Autodesk Fusion 360 part; units mm, degrees
(part 2 of 2)
sketch "Sketch11" plane through (0, 6.5, 0) normal (0, 1, 0) x (-1, 0, 0)
  line L0 (-40.9, 0) -> (-40.9, -16)
  line L1 (-40.9, -16) -> (-23.901, -16)
  line L2 (-23.901, -16) -> (-16.75, -17.1541)
  line L3 (-16.75, -17.1541) -> (-16.75, -8)
  line L4 (-16.75, -8) -> (-16.75, 1.1541)
  line L5 (-16.75, 1.1541) -> (-23.901, 0)
  line L6 (-23.901, 0) -> (-40.9, 0)
  arc A0 (2.6304, -1.5907) -> (-7.7128, 2.6127) centre (-6, -8) ccw
  arc A1 (-7.7128, 2.6127) -> (-11.9178, 0.9745) centre (-6, -8) ccw
  arc A2 (-16.75, -8) -> (-7.7128, -18.6127) centre (-6, -8) ccw
  line L7 (-16.75, -8) -> (-16.75, -17.1541)
  line L8 (-16.75, -17.1541) -> (-7.7128, -18.6127)
  arc A3 (-7.7128, 2.6127) -> (-16.75, -8) centre (-6, -8) ccw
  line L9 (-7.7128, 2.6127) -> (-16.75, 1.1541)
  line L10 (-16.75, 1.1541) -> (-16.75, -8)
  line L11 (-63.1, -16) -> (-63.1, 0)
  line L12 (-63.1, 0) -> (-68.099, 0)
  line L13 (-68.099, 0) -> (-75.25, 1.1541)
  line L14 (-75.25, 1.1541) -> (-75.25, -8)
  line L15 (-75.25, -8) -> (-75.25, -17.1541)
  line L16 (-75.25, -17.1541) -> (-68.099, -16)
  line L17 (-68.099, -16) -> (-63.1, -16)
  arc A4 (-84.2872, -18.6127) -> (-75.25, -8) centre (-86, -8) ccw
  arc A5 (-84.2872, -18.6127) -> (-75.25, -8) centre (-86, -8) ccw
  line L18 (-84.2872, -18.6127) -> (-75.25, -17.1541)
  line L19 (-75.25, -17.1541) -> (-75.25, -8)
  arc A6 (-84.2872, -18.6127) -> (-84.2872, 2.6127) centre (-86, -8) ccw
  arc A7 (-84.2872, 2.6127) -> (-84.2872, -18.6127) centre (-86, -8) ccw
  circle A8 centre (-86, -8) radius 3
  arc A9 (-75.25, -8) -> (-84.2872, 2.6127) centre (-86, -8) ccw
  line L20 (-75.25, -8) -> (-75.25, 1.1541)
  line L21 (-75.25, 1.1541) -> (-84.2872, 2.6127)
  circle A10 centre (-52, -12) radius 1.75
  circle A11 centre (-52, -4) radius 1.75
  line L22 (-47.9, -16) -> (-47.9, 0)
  line L23 (-47.9, 0) -> (-56.1, 0)
  line L24 (-56.1, 0) -> (-56.1, -16)
  line L25 (-56.1, -16) -> (-47.9, -16)
  line L26 (-60.1, -16) -> (-56.1, -16)
  line L27 (-56.1, -16) -> (-56.1, 0)
  line L28 (-56.1, 0) -> (-60.1, 0)
  line L29 (-60.1, 0) -> (-60.1, -16)
  line L30 (-63.1, -16) -> (-60.1, -16)
  line L31 (-60.1, -16) -> (-60.1, 0)
  line L32 (-60.1, 0) -> (-63.1, 0)
  line L33 (-63.1, 0) -> (-63.1, -16)
  line L34 (-47.9, -16) -> (-43.9, -16)
  line L35 (-43.9, -16) -> (-43.9, 0)
  line L36 (-43.9, 0) -> (-47.9, 0)
  line L37 (-47.9, 0) -> (-47.9, -16)
  line L38 (-40.9, 0) -> (-43.9, 0)
  line L39 (-43.9, 0) -> (-43.9, -16)
  line L40 (-43.9, -16) -> (-40.9, -16)
  line L41 (-40.9, -16) -> (-40.9, 0)
  line L42 (-6, -8) -> (-86, -8) construction
  line L43 (-22.325, -4.5) -> (-35.325, -4.5)
  arc A12 (-35.325, -4.5) -> (-35.325, -11.5) centre (-35.325, -8) ccw
  line L44 (-35.325, -11.5) -> (-22.325, -11.5)
  arc A13 (-22.325, -11.5) -> (-22.325, -4.5) centre (-22.325, -8) ccw
  line L45 (-22.325, -8) -> (-35.325, -8) construction
  line L46 (-68.175, -4.5) -> (-70.175, -4.5)
  arc A14 (-70.175, -4.5) -> (-70.175, -11.5) centre (-70.175, -8) ccw
  line L47 (-70.175, -11.5) -> (-68.175, -11.5)
  arc A15 (-68.175, -11.5) -> (-68.175, -4.5) centre (-68.175, -8) ccw
  line L48 (-68.175, -8) -> (-70.175, -8) construction
  arc A16 (-3.2196, -12.4938) -> (-1.2418, -15.3184) centre (-1.985, -13.7341) ccw
  arc A17 (-3.7269, -6.0422) -> (-7.4664, -5.3828) centre (-6, -8) ccw
  arc A18 (-11.7648, -13.7648) -> (-9.9843, -11.9843) centre (-10.015, -13.7341) ccw
  arc A19 (-0.2352, -2.2352) -> (-2.0157, -4.0157) centre (-1.985, -2.2659) ccw
  arc A20 (-8.7804, -3.5062) -> (-10.7582, -0.6816) centre (-10.015, -2.2659) ccw
  circle A21 centre (-93, -8) radius 1.75
  circle A22 centre (-86, -1) radius 1.75
  circle A23 centre (-86, -15) radius 1.75
  circle A24 centre (-79, -8) radius 1.75
  line L49 (-8.7804, -3.5062) -> (-7.4664, -5.3828)
  line L50 (-3.7269, -6.0422) -> (-1.8503, -4.7281)
  arc A25 (-2.0157, -4.0157) -> (-1.8503, -4.7281) centre (-0.2659, -3.985) ccw
  arc A26 (0.9743, -2.7503) -> (-0.2352, -2.2352) centre (-0.2659, -3.985) ccw
  line L51 (0.9743, -2.7503) -> (2.6304, -1.5907)
  line L52 (-11.9178, 0.9745) -> (-10.7582, -0.6816)
  arc A27 (-7.7128, -18.6127) -> (-0.0822, -16.9745) centre (-6, -8) ccw
  line L53 (-0.0822, -16.9745) -> (-1.2418, -15.3184)
  line L54 (-3.2196, -12.4938) -> (-4.5336, -10.6172)
  arc A28 (-8.2731, -9.9578) -> (-4.5336, -10.6172) centre (-6, -8) ccw
  line L55 (-8.2731, -9.9578) -> (-10.1497, -11.2719)
  arc A29 (-9.9843, -11.9843) -> (-10.1497, -11.2719) centre (-11.7341, -12.015) ccw
  arc A30 (-12.9743, -13.2497) -> (-11.7648, -13.7648) centre (-11.7341, -12.015) ccw
  line L56 (-12.9743, -13.2497) -> (-14.6304, -14.4093)
  arc A31 (-14.6304, -14.4093) -> (-7.7128, -18.6127) centre (-6, -8) ccw
  dimension "d45" = 13
  dimension "d46" = 3.5
  dimension "d47" = 24.15
  dimension "d48" = 5.575
  dimension "d49" = 3.5
  dimension "d50" = 2
  dimension "d51" = 12.15
  dimension "d52" = 5.075
  constraint coincident A0.centre A1.centre
  constraint coincident A4.centre A5.centre
  constraint tangent L43 A12
  constraint tangent A12 L44
  constraint parallel L43 L44
  constraint tangent L44 A13
  constraint tangent L43 A13
  constraint coincident L42 A12.centre
  constraint parallel L42 L45
  constraint tangent L46 A14
  constraint tangent A14 L47
  constraint parallel L46 L47
  constraint tangent L47 A15
  constraint tangent L46 A15
  constraint coincident L42 A14.centre
  constraint perpendicular L22 L48
  measures "d45" distance of A13.centre A12.centre
  measures "d46" distance of A13.centre L44
  measures "d47" distance of L10 L41
  measures "d48" distance of L4 A13.centre
  measures "d49" distance of A15.centre L46
  measures "d50" distance of A15.centre A14.centre
  measures "d51" distance of L11 L20
  measures "d52" distance of L14.end A14.centre
extrude "Extrude11" cut sketch "Sketch11" against normal up to surface (6.5 mm away) contours L43 A12 L44 A13 | L46 A14 L47 A15
fillet "Fillet1" radius 0.5 8 edges at (28.825, 6.5, -4.5) (18.825, 6.5, -8) (28.825, 6.5, -11.5) (38.825, 6.5, -8) (69.175, 6.5, -4.5) (64.675, 6.5, -8) (69.175, 6.5, -11.5) (73.675, 6.5, -8)
chamfer "Chamfer2" distance 0.5 angle 45 18 edges at (20.3255, 6.5, 0.5771) (32.4005, 6.5, 0) (42.4, 8, 0) (45.9, 9.5, 0) (47.9, 9.5, -8) (45.9, 9.5, -16) (42.4, 8, -16) (32.4005, 6.5, -16) (20.3255, 6.5, -16.5771) (56.1, 9.5, -8) (58.1, 9.5, 0) (61.6, 8, 0) (65.5995, 6.5, 0) (71.6745, 6.5, 0.5771) (71.6745, 6.5, -16.5771) (65.5995, 6.5, -16) (61.6, 8, -16) (58.1, 9.5, -16)
chamfer "Chamfer3" distance 0.5 angle 45 6 edges at (47.9, 7.5, 0) (52, 6, 0) (56.1, 7.5, 0) (47.9, 7.5, -16) (52, 6, -16) (56.1, 7.5, -16)
chamfer "Chamfer4" distance 0.5 angle 45 8 edges at (46, 0, 0) (15.8069, 0, 1.3063) (15.8069, 0, -17.3063) (-4.75, 0, -8) (46, 0, -16) (76.1931, 0, 1.3063) (76.1931, 0, -17.3063) (96.75, 0, -8)
equation "d30 = d29 / 2"
equation "d39 = d38"
equation "d41 = d42 / 4"
equation "d48 = ( d47 - d45 ) / 2"
equation "d49 = d46"
equation "d52 = ( d51 - d50 ) / 2"
equation "d65 = d60"
equation "d66 = d61"

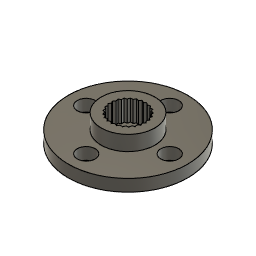
design "25TServoHorn"
Autodesk Fusion 360 part; units mm, degrees
sketch "Sketch1" plane through (0, 0, 0) normal (0, 1, 0) x (1, 0, 0)
  circle A0 centre (0, 0) radius 10
  circle A1 centre (0, 0) radius 4.5
  circle A2 centre (0, 0) radius 2.75
  circle A3 centre (0, 0) radius 1.5
  dimension "d1" = 20
  dimension "d2" = 9
  dimension "d3" = 5.5
  dimension "d4" = 3
  constraint coincident A0.centre A1.centre
  constraint concentric A1 A2
  measures "d1" diameter of A0
  measures "d2" diameter of A1
  measures "d3" diameter of A2
  measures "d4" diameter of A3
extrude "Extrude1" add sketch "Sketch1" along normal blind 2 contours A0
extrude "Extrude2" add sketch "Sketch1" along normal blind 4.5 contours A1
extrude "Extrude3" add sketch "Sketch1" along normal blind 1 contours A2
sketch "Sketch2" plane through (0, 2, 0) normal (0, 1, 0) x (-1, 0, 0)
  circle A0 centre (0, 0) radius 4.5
  circle A1 centre (0, 0) radius 10
  circle A2 centre (0, 0) radius 7
  circle A3 centre (7, 0) radius 1.5
  line L0 (0, 0) -> (10, 0) construction
  dimension "d11" = 14
  dimension "d12" = 3
  constraint concentric A0 A2
  constraint coincident A2 A3.centre
  constraint coincident A0.centre A1.centre
  constraint coincident A1 L0.end
  constraint horizontal L0
  constraint coincident A3.centre L0
  measures "d11" diameter of A2
  measures "d12" diameter of A3
extrude "Extrude4" cut sketch "Sketch2" against normal up to surface (2 mm away) contours A2 A3 | A2 A3 picked at (6.5153, -0.3111) picked at (7.4507, -0.3705)
pattern_circular "C-Pattern1" count 4 over 360 about axis through (0, 1.75, 0) along (0, 1, 0) of "Extrude4"
sketch "Sketch3" plane through (0, 4.5, 0) normal (0, 1, 0) x (-1, 0, 0)
  circle A0 centre (0, 0) radius 2.75
  circle A1 centre (0, 0) radius 4.5
  circle A2 centre (0, 0) radius 3
  line L0 (0, 0) -> (3, 0)
  line L1 (0, 0) -> (2.9763, -0.376)
  line L2 (0, 0) -> (2.9057, -0.7461)
  line L3 (2.6636, -0.6839) -> (2.9763, -0.376)
  line L4 (2.75, 0) -> (2.9763, -0.376)
  dimension "d17" = 6
  dimension "d18" = 7.2
  dimension "d19" = 14.4
  constraint concentric A0 A2
  constraint coincident A0.centre A1.centre
  constraint coincident A2 L0.end
  constraint horizontal L0
  constraint coincident A2 L1.end
  constraint coincident A2 L2.end
  constraint coincident L2 L3.start
  constraint coincident A0 L3.start
  constraint coincident L0 L4.start
  constraint coincident A0 L4.start
  measures "d17" diameter of A2
  measures "d18" angle of L0 L1
  measures "d19" angle of L0 L2
extrude "Extrude5" cut sketch "Sketch3" against normal up to surface (3.5 mm away) contours A0 L1 L4 | A0 L1 L3
pattern_circular "C-Pattern2" count 25 over 360 about axis through (0, 1.75, 0) along (0, 1, 0) of "Extrude5"

design "FrameSideServoHolder"
Autodesk Fusion 360 part; units mm, degrees
sketch "Sketch1" plane through (0, 0, 0) normal (0, 1, 0) x (1, 0, 0)
  line L0 (0, 0) -> (0, 7)
  line L1 (0, 7) -> (19, 7)
  line L2 (19, 7) -> (19, 48)
  line L3 (19, 48) -> (0, 48)
  line L4 (0, 48) -> (0, 55)
  line L5 (0, 55) -> (25, 55)
  line L6 (25, 55) -> (25, 34.5)
  line L7 (25, 34.5) -> (34.8, 24.7)
  line L8 (34.8, 24.7) -> (34.8, -3.9005)
  line L9 (34.8, -3.9005) -> (29.8503, -8.8503)
  line L10 (0, 0) -> (21, 0)
  line L11 (21, 0) -> (29.8503, -8.8503)
  line L12 (0, 7) -> (23.8995, 7) construction
  line L13 (23.8995, 7) -> (34.8, -3.9005) construction
  dimension "d1" = 7
  dimension "d2" = 7
  dimension "d3" = 19
  dimension "d4" = 41
  dimension "d5" = 135
  dimension "d6" = 6
  dimension "d7" = 20.5
  dimension "d8" = 15.8
  dimension "d9" = 135
  dimension "d10" = 7
  dimension "d11" = 2
  dimension "d12" = 7
  constraint coincident L0.start L10.start
  constraint vertical L0
  constraint perpendicular L0 L1
  constraint perpendicular L1 L2
  constraint perpendicular L0 L3
  constraint perpendicular L3 L4
  constraint perpendicular L4 L5
  constraint perpendicular L5 L6
  constraint vertical L8
  constraint perpendicular L0 L10
  constraint collinear L0 L4
  constraint perpendicular L9 L11
  constraint coincident L0 L1.start
  constraint perpendicular L0 L12
  constraint parallel L11 L13
  measures "d1" distance of L0.start L0.end
  measures "d2" distance of L3.end L4.end
  measures "d3" distance of L2 L4
  measures "d4" distance of L1.end L2.end
  measures "d5" angle of L6 L7
  measures "d6" distance of L2 L6
  measures "d7" distance of L5.end L6.end
  measures "d8" distance of L2 L8
  measures "d9" angle of L10 L11
  measures "d10" distance of L8.end L9.end
  measures "d11" distance of L2 L10.end
  measures "d12" distance of L10 L12
extrude "Extrude1" add sketch "Sketch1" along normal blind 16
sketch "Sketch2" plane through (0, 16, 0) normal (0, 1, 0) x (-1, 0, 0)
  line L0 (0, 0) -> (-21, 0)
  line L1 (-21, 0) -> (-29.8503, 8.8503)
  line L2 (-29.8503, 8.8503) -> (-34.8, 3.9005)
  line L3 (-34.8, 3.9005) -> (-34.8, -24.7)
  line L4 (-34.8, -24.7) -> (-25, -34.5)
  line L5 (-25, -34.5) -> (-25, -55)
  line L6 (-25, -55) -> (0, -55)
  line L7 (0, -55) -> (0, -48)
  line L8 (0, -48) -> (-19, -48)
  line L9 (-19, -48) -> (-19, -7)
  line L10 (-19, -7) -> (0, -7)
  line L11 (0, -7) -> (0, 0)
  line L12 (-4.5, -51.5) -> (-14.5, -51.5) construction
  line L13 (-14.5, -51.5) -> (-14.5, -3.5) construction
  line L14 (-14.5, -3.5) -> (-4.5, -3.5) construction
  line L15 (-4.5, -3.5) -> (-4.5, -51.5) construction
  circle A0 centre (-4.5, -51.5) radius 1.75
  circle A1 centre (-14.5, -51.5) radius 1.75
  circle A2 centre (-14.5, -3.5) radius 1.75
  circle A3 centre (-4.5, -3.5) radius 1.75
  dimension "d15" = 10
  dimension "d16" = 48
  dimension "d17" = 19
  dimension "d18" = 55
  dimension "d19" = 3.5
  dimension "d20" = 4.5
  dimension "d21" = 3.5
  dimension "d22" = 3.5
  dimension "d23" = 3.5
  dimension "d24" = 3.5
  constraint horizontal L12
  constraint vertical L13
  constraint horizontal L14
  constraint vertical L15
  constraint coincident L12.start L15.end
  constraint coincident L12.end L13.start
  constraint coincident L13.end L14.start
  constraint coincident L14.end L15.start
  measures "d15" distance of L12.start L12.end
  measures "d16" distance of L12.start L14.end
  measures "d17" distance of L7 L9
  measures "d18" distance of L0 L6
  measures "d19" distance of L6 L12
  measures "d20" distance of L7 L15
  measures "d21" diameter of A0
  measures "d22" diameter of A1
  measures "d23" diameter of A3
  measures "d24" diameter of A2
extrude "Extrude2" cut sketch "Sketch2" against normal up to surface (16 mm away) contours A0 | A1 | A2 | A3
sketch "Sketch3" plane through (0, 16, 0) normal (0, 1, 0) x (-1, 0, 0)
  circle A0 centre (-14.5, -51.5) radius 1.75
  circle A1 centre (-4.5, -3.5) radius 1.75
  circle A2 centre (-4.5, -51.5) radius 1.75
  circle A3 centre (-14.5, -3.5) radius 1.75
  line L0 (0, 0) -> (-21, 0)
  line L1 (-21, 0) -> (-29.8503, 8.8503)
  line L2 (-29.8503, 8.8503) -> (-34.8, 3.9005)
  line L3 (-34.8, 3.9005) -> (-34.8, -24.7)
  line L4 (-34.8, -24.7) -> (-25, -34.5)
  line L5 (-25, -34.5) -> (-25, -55)
  line L6 (-25, -55) -> (0, -55)
  line L7 (0, -55) -> (0, -48)
  line L8 (0, -48) -> (-19, -48)
  line L9 (-19, -48) -> (-19, -7)
  line L10 (-19, -7) -> (0, -7)
  line L11 (0, -7) -> (0, 0)
  line L12 (-25, -28.8431) -> (-30.8, -23.0431)
  line L13 (-25, -5.8995) -> (-25, -28.8431)
  line L14 (-30.8, -23.0431) -> (-30.8, -0.0995)
  line L15 (-30.8, -0.0995) -> (-25, -5.8995)
  dimension "d27" = 4
  dimension "d31" = 4
  dimension "d32" = 7
  constraint parallel L4 L12
  constraint parallel L9 L13
  constraint collinear L5 L13
  constraint parallel L3 L14
  constraint parallel L1 L15
  measures "d27" distance of L4 L12
  measures "d31" distance of L3 L14
  measures "d32" distance of L1 L15
extrude "Extrude3" cut sketch "Sketch3" against normal up to surface (16 mm away) contours L12 L13 L14 L15
sketch "Sketch4" plane through (0, 0, -55) normal (0, 0, -1) x (-1, 0, 0)
  line L0 (-25, 0) -> (0, 0)
  line L1 (0, 0) -> (0, 16)
  line L2 (0, 16) -> (-25, 16)
  line L3 (-25, 16) -> (-25, 0)
  line L4 (-34.8, 0) -> (-25, 0)
  line L5 (-25, 0) -> (-25, 16)
  line L6 (-25, 16) -> (-34.8, 16)
  line L7 (-34.8, 16) -> (-34.8, 0)
  line L8 (-25, 3) -> (-30, 3)
  line L9 (-30, 3) -> (-30, 13)
  line L10 (-30, 13) -> (-25, 13)
  line L11 (-25, 13) -> (-25, 3)
  dimension "d35" = 5
  dimension "d36" = 10
  dimension "d37" = 16
  dimension "d38" = 3
  constraint horizontal L8
  constraint vertical L9
  constraint horizontal L10
  constraint vertical L11
  constraint coincident L3 L8.start
  measures "d35" distance of L8.start L8.end
  measures "d36" distance of L8.end L9.end
  measures "d37" distance of L4.start L6.end
  measures "d38" distance of L4 L8
extrude "Extrude4" cut sketch "Sketch4" along normal up to surface contours L3 L5 L8 L9 L10 L11 end surface through (25, 16, -28.8431) normal (-0.707107, 0, 0.707107) offset 0
ref_plane "WorkPlane1" through (17.4, 8, -23.0749) normal (0, -1, 0) x (-1, 0, 0)
ref_plane "WorkPlane2" through (10.5, 8, -27.5) normal (0, 0, 1) x (1, 0, 0)
sketch "Sketch5" plane through (17.4, 8, -23.0749) normal (0, -1, 0) x (1, 0, 0)
  line L0 (13.4, 22.9754) -> (7.6, 17.1754)
  line L1 (7.6, 17.1754) -> (7.6, -5.7683)
  line L2 (7.6, -5.7683) -> (13.4, 0.0317)
  line L3 (13.4, 0.0317) -> (13.4, 22.9754)
  circle A0 centre (-2.9, -28.4251) radius 1.75
  circle A1 centre (-12.9, 19.5749) radius 1.75
  circle A2 centre (-12.9, -28.4251) radius 1.75
  circle A3 centre (-2.9, 19.5749) radius 1.75
  line L4 (-17.4, 23.0749) -> (3.6, 23.0749)
  line L5 (3.6, 23.0749) -> (12.4503, 31.9251)
  line L6 (12.4503, 31.9251) -> (17.4, 26.9754)
  line L7 (17.4, 26.9754) -> (17.4, -1.6251)
  line L8 (17.4, -1.6251) -> (7.6, -11.4251)
  line L9 (7.6, -11.4251) -> (7.6, -31.9251)
  line L10 (7.6, -31.9251) -> (-17.4, -31.9251)
  line L11 (-17.4, -31.9251) -> (-17.4, -24.9251)
  line L12 (-17.4, -24.9251) -> (1.6, -24.9251)
  line L13 (1.6, -24.9251) -> (1.6, 16.0749)
  line L14 (1.6, 16.0749) -> (-17.4, 16.0749)
  line L15 (-17.4, 16.0749) -> (-17.4, 23.0749)
  line L16 (7.6, 17.1754) -> (4.4518, 23.9267)
  line L17 (-0.6679, 23.0749) -> (7.6, 5.3444)
  dimension "d48" = 5
  dimension "d49" = 65
  constraint coincident L0.end L1.start
  constraint coincident L5 L16.end
  constraint coincident L4 L17.start
  constraint coincident L1 L17.end
  constraint parallel L16 L17
  measures "d48" distance of L16 L17
  measures "d49" angle of L4 L17
extrude "Extrude5" cut sketch "Sketch5" along normal mid plane 10 contours L1 L4 L5 L16 L17
sketch "Sketch6" plane through (10.5, 0, -10.5) normal (-0.707107, 0, 0.707107) x (0.707107, 0, 0.707107)
  line L0 (16.0539, 3) -> (14.8492, 3)
  line L1 (14.8492, 3) -> (14.8492, 0)
  line L2 (14.8492, 0) -> (27.3654, 0)
  line L3 (27.3654, 0) -> (27.3654, 16)
  line L4 (27.3654, 16) -> (14.8492, 16)
  line L5 (14.8492, 16) -> (14.8492, 13)
  line L6 (14.8492, 13) -> (16.0539, 13)
  line L7 (16.0539, 13) -> (16.0539, 3)
  line L8 (21.7085, 0) -> (13.5061, 0)
  line L9 (13.5061, 0) -> (13.5061, 3)
  line L10 (13.5061, 3) -> (13.5061, 13)
  line L11 (13.5061, 13) -> (13.5061, 16)
  line L12 (13.5061, 16) -> (21.7085, 16)
  line L13 (21.7085, 16) -> (21.7085, 0)
  line L14 (21.1073, 16) -> (21.1073, 0) construction
  line L15 (27.3654, 8) -> (13.5061, 8) construction
  circle A0 centre (21.1073, 8) radius 1.75
  dimension "d50" = 3.5
  constraint midpoint L4 L14.start
  constraint midpoint L2 L14.end
  constraint midpoint L3 L15.start
  constraint midpoint L10 L15.end
  constraint midpoint L14 A0.centre
  measures "d50" diameter of A0
extrude "Extrude6" cut sketch "Sketch6" against normal up to surface (7 mm away) contours L13 A0 | L13 A0
sketch "Sketch7" plane through (15.4497, 0, -15.4497) normal (0.707107, 0, -0.707107) x (-0.707107, 0, -0.707107)
  arc A0 (-21.7085, 6.3565) -> (-21.7085, 9.6435) centre (-21.1073, 8) ccw
  line L0 (-21.7085, 6.3565) -> (-21.7085, 0)
  line L1 (-21.7085, 0) -> (-13.5061, 0)
  line L2 (-13.5061, 0) -> (-13.5061, 3)
  line L3 (-13.5061, 3) -> (-13.5061, 13)
  line L4 (-13.5061, 13) -> (-13.5061, 16)
  line L5 (-13.5061, 16) -> (-21.7085, 16)
  line L6 (-21.7085, 16) -> (-21.7085, 9.6435)
  line L7 (-27.3654, 0) -> (-7.1418, 0)
  line L8 (-7.1418, 0) -> (-7.1418, 16)
  line L9 (-7.1418, 16) -> (-27.3654, 16)
  line L10 (-27.3654, 16) -> (-27.3654, 0)
  circle A1 centre (-21.1073, 8) radius 1.75
  circle A2 centre (-21.1073, 8) radius 3
  dimension "d53" = 6
  constraint concentric A0 A2
  measures "d53" diameter of A2
extrude "Extrude7" cut sketch "Sketch7" along normal up to surface contours A0 A1 | A0 L0 L6 A1 A2 | L0 L6 A1 A2 end surface through (34.8, 0, -24.7) normal (1, 0, 0) offset 0
sketch "Sketch8" plane through (17.4, 8, -23.0749) normal (0, -1, 0) x (1, 0, 0)
  line L0 (13.4, 22.9754) -> (7.6, 17.1754)
  line L1 (7.6, 17.1754) -> (7.6, -5.7683)
  line L2 (7.6, -5.7683) -> (13.4, 0.0317)
  line L3 (13.4, 0.0317) -> (13.4, 22.9754)
  circle A0 centre (-2.9, -28.4251) radius 1.75
  circle A1 centre (-12.9, 19.5749) radius 1.75
  circle A2 centre (-12.9, -28.4251) radius 1.75
  circle A3 centre (-2.9, 19.5749) radius 1.75
  line L4 (-17.4, 23.0749) -> (3.6, 23.0749)
  line L5 (3.6, 23.0749) -> (12.4503, 31.9251)
  line L6 (12.4503, 31.9251) -> (17.4, 26.9754)
  line L7 (17.4, 26.9754) -> (17.4, -1.6251)
  line L8 (17.4, -1.6251) -> (7.6, -11.4251)
  line L9 (7.6, -11.4251) -> (7.6, -31.9251)
  line L10 (7.6, -31.9251) -> (-17.4, -31.9251)
  line L11 (-17.4, -31.9251) -> (-17.4, -24.9251)
  line L12 (-17.4, -24.9251) -> (1.6, -24.9251)
  line L13 (1.6, -24.9251) -> (1.6, 16.0749)
  line L14 (1.6, 16.0749) -> (-17.4, 16.0749)
  line L15 (-17.4, 16.0749) -> (-17.4, 23.0749)
  line L16 (-10.2, 21.1337) -> (-12.9, 22.6926)
  line L17 (-12.9, 22.6926) -> (-15.6, 21.1337)
  line L18 (-15.6, 21.1337) -> (-15.6, 18.016)
  line L19 (-15.6, 18.016) -> (-12.9, 16.4572)
  line L20 (-12.9, 16.4572) -> (-10.2, 18.016)
  line L21 (-10.2, 18.016) -> (-10.2, 21.1337)
  line L22 (-0.2, 21.1337) -> (-2.9, 22.6926)
  line L23 (-2.9, 22.6926) -> (-5.6, 21.1337)
  line L24 (-5.6, 21.1337) -> (-5.6, 18.016)
  line L25 (-5.6, 18.016) -> (-2.9, 16.4572)
  line L26 (-2.9, 16.4572) -> (-0.2, 18.016)
  line L27 (-0.2, 18.016) -> (-0.2, 21.1337)
  line L28 (-15.6, 18.016) -> (-15.6, 16.0749)
  line L29 (-10.2, 18.016) -> (-10.2, 16.0749)
  line L30 (-15.6, 21.1337) -> (-15.6, 23.0749)
  line L31 (-10.2, 21.1337) -> (-10.2, 23.0749)
  line L32 (-5.6, 21.1337) -> (-5.6, 23.0749)
  line L33 (-0.2, 21.1337) -> (-0.2, 23.0749)
  line L34 (-5.6, 18.016) -> (-5.6, 16.0749)
  line L35 (-0.2, 18.016) -> (-0.2, 16.0749)
  point P0 (-12.9, 19.5749)
  point P1 (-2.9, 19.5749)
  dimension "d56" = 5.4
  dimension "d57" = 5.4
  constraint coincident P0 A1.centre
  constraint coincident P1 A3.centre
  constraint parallel L15 L18
  constraint parallel L21 L24
  constraint coincident L14 L28.end
  constraint perpendicular L14 L28
  constraint coincident L14 L29.end
  constraint perpendicular L14 L29
  constraint coincident L4 L30.end
  constraint perpendicular L4 L30
  constraint coincident L4 L31.end
  constraint perpendicular L4 L31
  constraint coincident L4 L32.end
  constraint perpendicular L4 L32
  constraint coincident L4 L33.end
  constraint perpendicular L4 L33
  constraint coincident L14 L34.end
  constraint perpendicular L14 L34
  constraint coincident L14 L35.end
  constraint perpendicular L14 L35
  measures "d56" distance of L18 L21
  measures "d57" distance of L24 L27
extrude "Extrude8" cut sketch "Sketch8" along normal mid plane 2.5 contours L4 L16 L17 L30 L31 | L16 L17 L18 L19 L20 L21 | L14 L19 L20 L28 L29 | L4 L22 L23 L32 L33 | L22 L23 L24 L25 L26 L27 | L14 L25 L26 L34 L35
mirror "Mirror1" about plane through (10.5, 8, -27.5) normal (0, 0, 1) of "Extrude8"
sketch "Sketch9" plane through (0, 0, 0) normal (0, 0, 1) x (1, 0, 0)
  line L0 (1.8, 9.25) -> (7.2, 9.25)
  line L1 (7.2, 9.25) -> (7.2, 6.75)
  line L2 (16.7321, 6.75) -> (11.8, 6.75)
  line L3 (1.8, 6.75) -> (1.8, 9.25)
  line L4 (11.8, 9.25) -> (16.7321, 9.25)
  line L5 (11.8, 6.75) -> (11.8, 9.25)
  line L6 (21, 3) -> (16.7321, 3)
  line L7 (16.7321, 9.25) -> (16.7321, 13)
  line L8 (16.7321, 13) -> (21, 13)
  line L9 (21, 13) -> (21, 16)
  line L10 (21, 16) -> (0, 16)
  line L11 (0, 16) -> (0, 0)
  line L12 (0, 0) -> (21, 0)
  line L13 (21, 0) -> (21, 3)
  line L14 (7.2, 9.25) -> (1.8, 9.25)
  line L15 (1.8, 9.25) -> (1.8, 6.75)
  line L16 (1.8, 6.75) -> (7.2, 6.75)
  line L17 (7.2, 6.75) -> (7.2, 9.25)
  line L18 (17.2, 9.25) -> (11.8, 9.25)
  line L19 (11.8, 9.25) -> (11.8, 6.75)
  line L20 (11.8, 6.75) -> (17.2, 6.75)
  line L21 (17.2, 6.75) -> (17.2, 9.25)
  line L22 (19, 0) -> (0, 0)
  line L23 (0, 0) -> (0, 16)
  line L24 (0, 16) -> (19, 16)
  line L25 (19, 16) -> (19, 0)
  line L26 (2.75, 16) -> (6.25, 16)
  line L27 (12.75, 16) -> (16.25, 16)
  line L28 (9.5, 16) -> (9.5, -0.0004) construction
  circle A0 centre (9.5, 12) radius 1.75
  circle A1 centre (9.5, 4) radius 1.75
  line L29 (16.7321, 3) -> (16.7321, 6.75)
  line L30 (7.2, 6.75) -> (1.8, 6.75)
  dimension "d60" = 19
  dimension "d61" = 9.5
  dimension "d62" = 3.5
  dimension "d63" = 3.5
  dimension "d64" = 4
  dimension "d65" = 4
  constraint vertical L28
  constraint coincident L24 L28.start
  constraint coincident L28 A0.centre
  constraint coincident L28 A1.centre
  measures "d60" distance of L11 L25
  measures "d61" distance of L23 L28
  measures "d62" diameter of A0
  measures "d63" diameter of A1
  measures "d64" distance of L24 A0.centre
  measures "d65" distance of L22 A1.centre
extrude "Extrude9" cut sketch "Sketch9" against normal up to surface (7 mm away) contours A0 | A1
sketch "Sketch10" plane through (0, 0, -7) normal (0, 0, -1) x (-1, 0, 0)
  circle A0 centre (-9.5, 12) radius 1.75
  circle A1 centre (-9.5, 4) radius 1.75
  line L0 (-7.2, 9.25) -> (-1.8, 9.25)
  line L1 (-1.8, 9.25) -> (-1.8, 6.75)
  line L2 (-1.8, 6.75) -> (-7.2, 6.75)
  line L3 (-7.2, 6.75) -> (-7.2, 9.25)
  line L4 (-17.2, 9.25) -> (-11.8, 9.25)
  line L5 (-11.8, 9.25) -> (-11.8, 6.75)
  line L6 (-11.8, 6.75) -> (-17.2, 6.75)
  line L7 (-17.2, 6.75) -> (-17.2, 9.25)
  line L8 (-19, 0) -> (0, 0)
  line L9 (0, 0) -> (0, 16)
  line L10 (0, 16) -> (-19, 16)
  line L11 (-19, 16) -> (-19, 0)
  circle A2 centre (-9.5, 12) radius 2.9
  circle A3 centre (-9.5, 4) radius 2.9
  dimension "d70" = 5.8
  dimension "d71" = 5.8
  constraint concentric A0 A2
  constraint concentric A1 A3
  measures "d70" diameter of A2
  measures "d71" diameter of A3
extrude "Extrude10" cut sketch "Sketch10" against normal blind 3 contours A2 | A3
sketch "Sketch11" plane through (0, 0, -55) normal (0, 0, -1) x (-1, 0, 0)
  line L0 (-7.2, 9.25) -> (-1.8, 9.25)
  line L1 (-1.8, 9.25) -> (-1.8, 6.75)
  line L2 (-1.8, 6.75) -> (-7.2, 6.75)
  line L3 (-7.2, 6.75) -> (-7.2, 9.25)
  line L4 (-17.2, 9.25) -> (-11.8, 9.25)
  line L5 (-11.8, 9.25) -> (-11.8, 6.75)
  line L6 (-11.8, 6.75) -> (-17.2, 6.75)
  line L7 (-17.2, 6.75) -> (-17.2, 9.25)
  line L8 (-25, 0) -> (0, 0)
  line L9 (0, 0) -> (0, 16)
  line L10 (0, 16) -> (-25, 16)
  line L11 (-25, 16) -> (-25, 0)
  circle A0 centre (-9.5, 12) radius 2.9
  circle A1 centre (-9.5, 4) radius 2.9
  line L12 (-7.2, 9.25) -> (-1.8, 9.25)
  line L13 (-1.8, 9.25) -> (-1.8, 6.75)
  line L14 (-1.8, 6.75) -> (-7.2, 6.75)
  line L15 (-7.2, 6.75) -> (-7.2, 9.25)
  line L16 (-17.2, 9.25) -> (-11.8, 9.25)
  line L17 (-11.8, 9.25) -> (-11.8, 6.75)
  line L18 (-11.8, 6.75) -> (-17.2, 6.75)
  line L19 (-17.2, 6.75) -> (-17.2, 9.25)
  line L20 (-19, 0) -> (0, 0)
  line L21 (0, 0) -> (0, 16)
  line L22 (0, 16) -> (-19, 16)
  line L23 (-19, 16) -> (-19, 0)
  circle A2 centre (-9.5, 12) radius 1.75
  circle A3 centre (-9.5, 4) radius 1.75
  circle A4 centre (-9.5, 12) radius 2.5
  circle A5 centre (-9.5, 4) radius 2.5
  dimension "d74" = 5
  dimension "d75" = 5
  constraint concentric A0 A4
  constraint concentric A3 A5
  measures "d74" diameter of A4
  measures "d75" diameter of A5
extrude "Extrude11" cut sketch "Sketch11" against normal up to surface (7 mm away) contours A2 | A3 | A4 | A5
sketch "Sketch12" plane through (0, 0, -55) normal (0, 0, -1) x (-1, 0, 0)
  circle A0 centre (-9.5, 12) radius 2.5
  circle A1 centre (-9.5, 4) radius 2.5
  line L0 (-7.2, 9.25) -> (-1.8, 9.25)
  line L1 (-1.8, 9.25) -> (-1.8, 6.75)
  line L2 (-1.8, 6.75) -> (-7.2, 6.75)
  line L3 (-7.2, 6.75) -> (-7.2, 9.25)
  line L4 (-17.2, 9.25) -> (-11.8, 9.25)
  line L5 (-11.8, 9.25) -> (-11.8, 6.75)
  line L6 (-11.8, 6.75) -> (-17.2, 6.75)
  line L7 (-17.2, 6.75) -> (-17.2, 9.25)
  line L8 (-25, 0) -> (0, 0)
  line L9 (0, 0) -> (0, 16)
  line L10 (0, 16) -> (-25, 16)
  line L11 (-25, 16) -> (-25, 0)
  line L12 (-25, 3) -> (-30, 3)
  line L13 (-30, 3) -> (-30, 13)
  line L14 (-30, 13) -> (-25, 13)
  line L15 (-25, 13) -> (-25, 16)
  line L16 (-25, 16) -> (-34.8, 16)
  line L17 (-34.8, 16) -> (-34.8, 0)
  line L18 (-34.8, 0) -> (-25, 0)
  line L19 (-25, 0) -> (-25, 3)
  line L20 (-30.8, 5.0609) -> (-30.8, 0)
  line L21 (-30.8, 0) -> (-25, 0)
  line L22 (-25, 0) -> (-25, 3)
  line L23 (-25, 3) -> (-25, 13)
  line L24 (-25, 13) -> (-25, 16)
  line L25 (-25, 16) -> (-30.8, 16)
  line L26 (-30.8, 16) -> (-30.8, 10.9391)
  ellipse E0 centre (-30.3749, 8) end of major axis (-30.3749, 11) minor radius 2.1213 (-30.8, 10.9391) -> (-30.8, 5.0609) ccw
  ellipse E1 centre (-30.3749, 8) end of major axis (-30.3749, 9.75) minor radius 1.2374
  line L27 (-25, 3) -> (-23, 5)
  line L28 (-23, 5) -> (-23, 11)
  line L29 (-23, 11) -> (-25, 13)
  dimension "d82" = 45
  dimension "d83" = 45
  dimension "d84" = 2
  constraint coincident L12.start L19.end
  constraint parallel L11 L28
  constraint coincident L14.end L15.start
  measures "d82" angle of L23 L27
  measures "d83" angle of L11 L29
  measures "d84" distance of L11 L28
extrude "Extrude12" cut sketch "Sketch12" along normal up to surface contours L11 L23 L27 L28 L29 end surface through (16.7321, 8, 0) normal (0.906308, 0, 0.422618) offset 0
sketch "Sketch16" plane through (0, 0, -7) normal (0, 0, -1) x (-1, 0, 0)
  circle A0 centre (-9.5, 12) radius 2.9
  circle A1 centre (-9.5, 4) radius 2.9
  line L0 (-7.2, 9.25) -> (-1.8, 9.25)
  line L1 (-1.8, 9.25) -> (-1.8, 6.75)
  line L2 (-1.8, 6.75) -> (-7.2, 6.75)
  line L3 (-7.2, 6.75) -> (-7.2, 9.25)
  line L4 (-17.2, 9.25) -> (-11.8, 9.25)
  line L5 (-11.8, 9.25) -> (-11.8, 6.75)
  line L6 (-11.8, 6.75) -> (-17.2, 6.75)
  line L7 (-17.2, 6.75) -> (-17.2, 9.25)
  line L8 (-19, 0) -> (0, 0)
  line L9 (0, 0) -> (0, 16)
  line L10 (0, 16) -> (-19, 16)
  line L11 (-19, 16) -> (-19, 0)
  point P0 (0, 14)
  point P1 (-2, 16)
  dimension "d94" = 2
  dimension "d95" = 2
  constraint coincident L9 P0
  constraint coincident L10 P1
  measures "d94" distance of L9.end P0
  measures "d95" distance of L9.end P1
sketch "Sketch17" plane through (0, 0, 0) normal (-1, 0, 0) x (0, 0, 1)
  line L0 (-7, 0) -> (0, 0)
  line L1 (0, 0) -> (0, 16)
  line L2 (0, 16) -> (-7, 16)
  line L3 (-7, 16) -> (-7, 0)
  point P0 (-5, 16)
  point P1 (-7, 16)
  dimension "d96" = 2
  constraint coincident L2 P0
  measures "d96" distance of P0 P1
ref_plane "WorkPlane4" through (0, 14, -7) normal (0.57735, -0.57735, 0.57735) x (0.707107, 0.707107, 0)
sketch "Sketch18" plane through (0, 14, -7) normal (0.57735, -0.57735, 0.57735) x (0.707107, 0.707107, 0)
  line L0 (1.4142, 2.4495) -> (2.8284, 0)
  line L1 (2.8284, 0) -> (0, 0)
  line L2 (0, 0) -> (1.4142, 2.4495)
  point P0 (1.4142, 2.4495)
  point P1 (2.8284, 0)
  constraint coincident P0 L0.start
  constraint coincident P1 L0.end
  constraint coincident L1.end L2.start
extrude "Extrude14" cut sketch "Sketch18" against normal up to surface (1.1547 mm away)
mirror "Mirror3" about plane through (17.4, 8, -23.0749) normal (0, -1, 0) of "Extrude14"
chamfer "Chamfer1" distance 5 angle 45 2 edges at (25, 14.5, -55) (25, 1.5, -55)
chamfer "Chamfer2" distance 2 angle 45 10 edges at (32.3251, 16, 6.3754) (34.8, 16, -10.3997) (29.9, 16, -29.6) (25, 16, -42.25) (22.5, 16, -52.5) (22.5, 0, -52.5) (25, 0, -42.25) (29.9, 0, -29.6) (34.8, 0, -10.3997) (32.3251, 0, 6.3754)
chamfer "Chamfer3" distance 1.5 angle 45 8 edges at (30.8, 16, -11.5713) (27.9, 16, -2.9995) (25, 16, -17.3713) (27.9, 16, -25.9431) (27.9, 0, -25.9431) (30.8, 0, -11.5713) (25, 0, -17.3713) (27.9, 0, -2.9995)
chamfer "Chamfer4" distance 0.5 angle 45 19 edges at (29.8503, 8, 8.8503) (29.1431, 1, 8.1431) (24.718, 0, 3.718) (10.5, 0, 0) (0, 0, -3.5) (9.5, 0, -7) (19, 0, -27.5) (9.5, 0, -48) (0, 0, -51.5) (8.5858, 0, -55) (29.1431, 15, 8.1431) (24.718, 16, 3.718) (10.5, 16, 0) (0, 16, -3.5) (9.5, 16, -7) (19, 16, -27.5) (9.5, 16, -48) (0, 16, -51.5) (8.5858, 16, -55)
equation "d2 = d1"
equation "d12 = d10"
equation "d19 = ( d18 - d16 ) / 2"
equation "d20 = ( d17 - d15 ) / 2"
equation "d22 = d21"
equation "d23 = d21"
equation "d24 = d21"
equation "d38 = ( d37 - d36 ) / 2"
equation "d57 = d56"
equation "d61 = d60 / 2"
equation "d65 = d64"
equation "d71 = d70"
equation "d75 = d74"
equation "d95 = d94"
